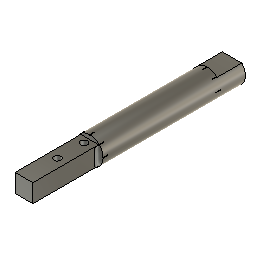
UCF_MainArm v3 (Autodesk Fusion 360 design; units mm, degrees)
Autodesk Fusion 360 part; units mm, degrees
sketch "Sketch1" plane through (0, 0, 0) normal (0, 1, 0) x (1, 0, 0)
  circle A0 centre (0, 0) radius 9.525
  line L0 (-6.35, -6.49224) -> (-6.35, 6.49224)
  line L1 (6.35, 6.49224) -> (6.35, -6.49224)
  line L2 (-6.96968, -6.49224) -> (6.96968, -6.49224)
  line L3 (6.96968, 6.49224) -> (-6.96968, 6.49224)
  circle A1 centre (0, 0) radius 12.7 construction
  dimension "d1" = 19.05
  dimension "d11" = 6.49224
  dimension "d12" = 6.49224
  dimension "d92" = 25.4
  dimension "d200" = 6.35
  dimension "d201" = 12.7
  constraint coincident A0.centre A1.centre
  constraint parallel L0 L1
  constraint perpendicular L1 L2
  constraint perpendicular L0 L3
  constraint concentric A0 A1
  constraint vertical L0
  measures "d1" diameter of A0
  measures "d11" distance of A0.centre L2
  measures "d12" distance of A0.centre L3
  measures "d92" diameter of A1
  measures "d200" distance of L0 A0.centre
  measures "d201" distance of L0 L1
extrude "Extrude1" add sketch "Sketch1" along normal blind 114.3 contours A0 L1 L2 L3 | A0 L3 | A0 L2 | A0 L0 L2 L3 | L0 L1 L2 L3 picked at (7.408333, 0) picked at (-0.236707, 7.494324) picked at (0.236707, -7.494324) picked at (-7.408333, 0) picked at (-2.116667, 2.16408)
extrude "Extrude2" cut sketch "Sketch1" against normal blind 12.7 from surface at 114.3 contours A0 L1 L2 L3 | A0 L3 | A0 L2 | A0 L0 L2 L3 | L0 L1 L2 L3 picked at (7.408333, 0) picked at (-0.236707, 7.494324) picked at (0.236707, -7.494324) picked at (-7.408333, 0) picked at (-2.116667, 2.16408)
extrude "Extrude3" add sketch "Sketch1" against normal blind 46.99 contours L0 L1 L2 L3 picked at (-2.116667, 2.16408)
sketch "Sketch2" plane through (0, 0, 6.49224) normal (0, 0, 1) x (-1, 0, 0)
  circle A0 centre (0, 23.114) radius 2.4892
  circle A1 centre (0, 4.064) radius 2.4892
  dimension "d25" = 4.9784
  dimension "d26" = 4.9784
  dimension "d27" = 19.05
  dimension "d413" = 4.064
  constraint vertical A0.centre A1.centre
  constraint vertical origin A1.centre
  measures "d25" diameter of A0
  measures "d26" diameter of A1
  measures "d27" distance of A0.centre A1.centre
  measures "d413" distance of origin A1.centre
extrude "Extrude4" cut sketch "Sketch2" against normal up to surface (12.98448 mm away) contours A0 | A1 picked at (-1.465566, 22.807799) picked at (0.986242, 5.102364)
extrude "Extrude5" cut sketch "Sketch1" against normal blind 17.78 from surface at 101.6 contours A0 L2 picked at (0.236707, -7.494324)
fillet "Fillet2" radius 3.175 2 edges at (-6.35, 0, 0) (6.35, 0, 0)
sketch "Sketch3" plane through (0, 0, 0) normal (0, 0, 1) x (1, 0, 0)
  line L0 (0, 0) -> (0, 3.175) construction
  line L1 (0.127, 0) -> (0.127, 3.175)
  line L2 (-0.127, 0) -> (-0.127, 3.175)
  line L3 (0.127, 3.175) -> (-0.127, 3.175)
  line L4 (0.127, 0) -> (0, 0)
  line L5 (0.127, 0) -> (-0.127, 0)
  dimension "d378" = 3.175
  dimension "d379" = 0.127
  constraint coincident L0.start L4.end
  constraint vertical L0
  constraint symmetric L0 L1.start L2.start
  constraint symmetric L0 L1.end L2.end
  constraint perpendicular L2 L4
  measures "d378" distance of L0.start L0.end
extrude "Extrude6" cut sketch "Sketch3" against normal blind 0.381 from the near side of the face at (-7.63025, 37.212514, -5.701307) contours L1 L2 L3 L4 L5 picked at (0, 2.116667)
pattern_circular "C-Pattern1" count 5 over 180 about axis through (0, 0, 0) along (0, 1, 0) both ways of "Extrude6"
ref_plane "WorkPlane2" through (0, 41.91, 0) normal (0, -1, 0) x (-1, 0, 0)
mirror "Mirror1" about plane through (0, 41.91, 0) normal (0, -1, 0) of "Extrude6", "C-Pattern1"
equation "d12 = d11"
equation "d26 = d25"
